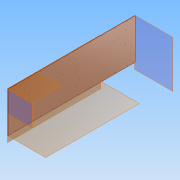
# Autodesk Inventor part: Top_Backboard
Saved by Autodesk Inventor 2018.1 (Build 221171000, 171)
## iProperties
Created: 2019-03-15
Part Number: Top_Backboard
Material: Wood (Oak)
Document SubType Name: Modeling
Designer: James
Density: 0.76 g/cm^3
Appearance: White Oak - Natural Medium Gloss
Author: James
Autodesk Inventor part; units mm, degrees
ref_plane "YZ Plane" through (0, 0, 0) normal (1, 0, 0) x (0, 1, 0)
ref_plane "XZ Plane" through (0, 0, 0) normal (0, 1, 0) x (-1, 0, 0)
ref_plane "XY Plane" through (0, 0, 0) normal (0, 0, 1) x (1, 0, 0)
derived "Top_Skeleton.ipt"
ref_plane "Work Plane1" through (0, 0, 0) normal (0, 0, 1) x (1, 0, 0)
ref_plane "Work Plane2" through (0, 0, 0) normal (0, 1, 0) x (-1, 0, 0)
ref_plane "Work Plane3" through (0, 0, 0) normal (1, 0, 0) x (0, 1, 0)
ref_plane "Work Plane4" through (0, 4100, 0) normal (0, 1, 0) x (-1, 0, 0)
ref_plane "Work Plane5" through (0, 0, -1300) normal (0, 0, 1) x (1, 0, 0)
sketch "Sketch2" plane through (0, 0, 0) normal (1, 0, 0) x (0, 1, 0)
  line L0 (0, 300) -> (0, -1800) projected
  line L1 (-820, 0) -> (4920, 0) projected
  line L2 (-820, -1300) -> (4920, -1300) projected
  line L3 (4100, 300) -> (4100, -1800) projected
  line L4 (0, 0) -> (4100, 0)
  line L5 (4100, 0) -> (4100, -1300)
  line L6 (4100, -1300) -> (0, -1300)
  line L7 (0, -1300) -> (0, 0)
  constraints: 8 end point, 4 point on line, 2 parallel, 1 horizontal, 1 perpendicular
extrude "Extrusion2" add sketch "Sketch2" along normal blind 15
sketch "Sketch3" plane through (15, 0, 0) normal (1, 0, 0) x (0, 0, -1)
  line L0 (1300, 4100) -> (0, 4100) projected
  line L1 (0, 4100) -> (0, 0) projected
  point P0 (487.5, 3991.5)
  point P1 (487.5, 3841.5)
  point P2 (822.5, 3841.5)
  point P3 (822.5, 3991.5)
  point P4 (487.5, 2881.3)
  point P5 (772.5, 2881.3)
  point P6 (772.5, 2731.3)
  point P7 (487.5, 2731.3)
  point P8 (487.5, 1771.1)
  point P9 (722.5, 1771.1)
  point P10 (722.5, 1621.1)
  point P11 (487.5, 1621.1)
  point P12 (487.5, 660.9)
  point P13 (672.5, 660.9)
  point P14 (672.5, 510.9)
  point P15 (487.5, 510.9)
  dimension "d7" = 150
  dimension "d8" = 335
  dimension "d16" = 150
  dimension "d17" = 150
  dimension "d18" = 150
  dimension "d19" = 285
  dimension "d20" = 235
  dimension "d21" = 185
  dimension "d22" = 108.5
  dimension "d23" = 487.5
  dimension "d24" = 1110.2
  dimension "d25" = 1110.2
  dimension "d26" = 1110.2
  constraints: 11 vertical alignment, 8 horizontal alignment
  measures "d7" distance of point (487.5, 3841.5) point (487.5, 3991.5)
  measures "d8" distance of point (822.5, 3991.5) point (487.5, 3991.5)
  measures "d16" distance of point (487.5, 2731.3) point (487.5, 2881.3)
  measures "d17" distance of point (487.5, 1621.1) point (487.5, 1771.1)
  measures "d18" distance of point (487.5, 510.9) point (487.5, 660.9)
  measures "d19" distance of point (772.5, 2881.3) point (487.5, 2881.3)
  measures "d20" distance of point (722.5, 1771.1) point (487.5, 1771.1)
  measures "d21" distance of point (672.5, 660.9) point (487.5, 660.9)
  measures "d22" distance from line of L0 point (487.5, 3991.5)
  measures "d23" distance from line of L1 point (487.5, 3991.5)
  measures "d24" vertical distance of point (772.5, 2881.3) point (822.5, 3991.5)
  measures "d25" vertical distance of point (722.5, 1771.1) point (772.5, 2881.3)
  measures "d26" vertical distance of point (672.5, 660.9) point (722.5, 1771.1)
hole "Selection Holes" at (15, 3991.5, -487.5) at (15, 3841.5, -487.5) at (15, 3841.5, -822.5) at (15, 3991.5, -822.5) at (15, 2881.3, -772.5) at (15, 2731.3, -772.5) at (15, 2731.3, -487.5) at (15, 2881.3, -487.5) at (15, 1771.1, -487.5) at (15, 1621.1, -487.5) at (15, 1621.1, -722.5) at (15, 1771.1, -722.5) at (15, 660.9, -487.5) at (15, 660.9, -672.5) at (15, 510.9, -672.5) at (15, 510.9, -487.5) direction (-1, 0, 0) diameter 4.5 end through all clearance for "Flat Head Machine Screw" size "M4" standard "Ansi Metric M Profile"
sketch "Sketch4" plane through (15, 0, 0) normal (1, 0, 0) x (0, 0, -1)
  circle A0 centre (672.5, 510.9) radius 2.25 projected
  circle A1 centre (487.5, 660.9) radius 2.25 projected
  circle A2 centre (722.5, 1621.1) radius 2.25 projected
  circle A3 centre (487.5, 1771.1) radius 2.25 projected
  circle A4 centre (487.5, 2731.3) radius 2.25 projected
  circle A5 centre (772.5, 2881.3) radius 2.25 projected
  circle A6 centre (822.5, 3841.5) radius 2.25 projected
  circle A7 centre (487.5, 3991.5) radius 2.25 projected
  circle A8 centre (487.5, 3841.5) radius 2.25 projected
  circle A9 centre (822.5, 3991.5) radius 2.25 projected
  circle A10 centre (772.5, 2731.3) radius 2.25 projected
  circle A11 centre (487.5, 2881.3) radius 2.25 projected
  circle A12 centre (487.5, 1621.1) radius 2.25 projected
  circle A13 centre (722.5, 1771.1) radius 2.25 projected
  circle A14 centre (672.5, 660.9) radius 2.25 projected
  circle A15 centre (487.5, 510.9) radius 2.25 projected
  line L0 (0, 0) -> (1300, 0) projected
  line L1 (1300, 0) -> (1300, 4100) projected
  line L2 (1300, 4100) -> (0, 4100) projected
  line L3 (0, 4100) -> (0, 0) projected
  point P0 (380, 3563)
  point P1 (935, 3563)
  point P2 (935, 3413)
  point P3 (380, 3413)
  point P4 (425, 2452.5)
  point P5 (885, 2452.5)
  point P6 (885, 2302.5)
  point P7 (425, 2302.5)
  point P8 (470, 1342.5)
  point P9 (835, 1342.5)
  point P10 (835, 1192.5)
  point P11 (470, 1192.5)
  dimension "d27" = 150
  dimension "d28" = 150
  dimension "d29" = 150
  dimension "d30" = 380
  dimension "d31" = 425
  dimension "d32" = 470
  dimension "d33" = 460
  dimension "d34" = 365
  dimension "d35" = 555
  dimension "d43" = 537
  dimension "d49" = 1110.5
  dimension "d50" = 1110
  constraints: 6 horizontal alignment, 6 vertical alignment
  measures "d27" distance of point (835, 1192.5) point (835, 1342.5)
  measures "d28" distance of point (885, 2452.5) point (885, 2302.5)
  measures "d29" distance of point (935, 3563) point (935, 3413)
  measures "d30" distance from line of L3 point (380, 3563)
  measures "d31" distance from line of point (425, 2452.5) L3
  measures "d32" distance from line of point (470, 1342.5) L3
  measures "d33" distance of point (885, 2452.5) point (425, 2452.5)
  measures "d34" distance of point (835, 1342.5) point (470, 1342.5)
  measures "d35" distance of point (935, 3563) point (380, 3563)
  measures "d43" distance from line of L2 point (935, 3563)
  measures "d49" vertical distance of point (885, 2452.5) point (935, 3563)
  measures "d50" vertical distance of point (835, 1342.5) point (885, 2452.5)
hole "Pancake Holes" at (15, 3563, -380) at (15, 3563, -935) at (15, 3413, -935) at (15, 3413, -380) at (15, 2452.5, -425) at (15, 2452.5, -885) at (15, 2302.5, -885) at (15, 2302.5, -425) at (15, 1342.5, -470) at (15, 1342.5, -835) at (15, 1192.5, -835) at (15, 1192.5, -470) direction (-1, 0, 0) diameter 4.5 end through all clearance for "Flat Head Machine Screw" size "M4" standard "Ansi Metric M Profile"
pattern_linear "Rectangular Pattern1" count 2 spacing 250 along (0, -1, 0) of "Pancake Holes"
sketch "Sketch5" plane through (15, 0, 0) normal (1, 0, 0) x (0, 0, -1)
  line L0 (1300, 0) -> (1300, 4100) projected
  line L1 (0, 4100) -> (0, 0) projected
  line L2 (-260, 4100) -> (1560, 4100) projected
  point P0 (25, 3850)
  point P1 (1275, 3850)
  dimension "d51" = 25
  dimension "d52" = 25
  dimension "d53" = 250
  constraints: 1 horizontal alignment
  measures "d51" distance from line of L0 point (1275, 3850)
  measures "d52" distance from line of L1 point (25, 3850)
  measures "d53" distance from line of point (25, 3850) L2
hole "Hole3" at (15, 3850, -25) at (15, 3850, -1275) direction (-1, 0, 0) diameter 4.496 end through all countersink diameter 8.433 countersink angle 82 clearance for "Flat Head Machine Screw (82)" size "#8" standard "Ansi Unified Screw Threads"
pattern_linear "Rectangular Pattern2" count 10 spacing 400 along (0, -1, 0) of "Hole3"
sketch "Sketch6" plane through (15, 0, 0) normal (1, 0, 0) x (0, 0, -1)
  line L0 (0, 4100) -> (0, 0) projected
  line L1 (-260, 4100) -> (1560, 4100) projected
  point P0 (250, 3800)
  point P1 (250, 2170)
  point P2 (250, 540)
  dimension "d64" = 250
  dimension "d65" = 300
  dimension "d76" = 1630
  dimension "d77" = 1630
  constraints: 2 vertical alignment
  measures "d64" distance from line of point (250, 3800) L0
  measures "d65" distance from line of point (250, 3800) L1
  measures "d76" distance of point (250, 2170) point (250, 3800)
  measures "d77" distance of point (250, 540) point (250, 2170)
hole "Hole4" at (15, 3800, -250) at (15, 2170, -250) at (15, 540, -250) direction (-1, 0, 0) diameter 4.496 end through all countersink diameter 8.433 countersink angle 82 clearance for "Flat Head Machine Screw (82)" size "#8" standard "Ansi Unified Screw Threads"
pattern_linear "Rectangular Pattern3" count 3 spacing 400 along (0, 0, -1) of "Hole4"
equation "\"d16\" = d7"
equation "\"d17\" = d16"
equation "\"d18\" = d17"
equation "\"d25\" = d24"
equation "\"d26\" = d24"
equation "\"d28\" = d27"
equation "\"d29\" = d28"
equation "\"d52\" = d51"
equation "\"d77\" = d76"
body "Solid2"
